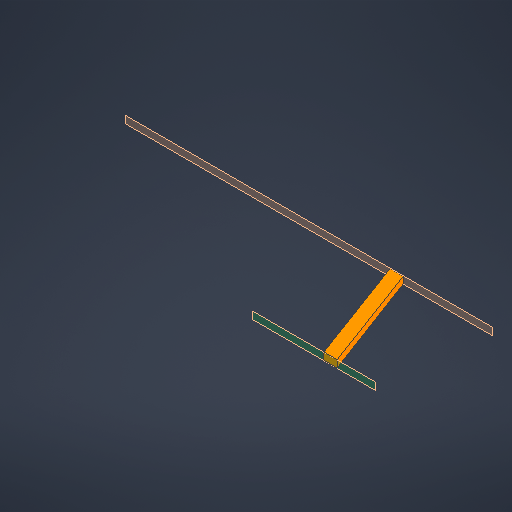
# Autodesk Inventor part: Renamev2
Saved by Autodesk Inventor 2027 (Build 310192000, 192)
## iProperties
Created: 2026-08-07
Part Number: Renamev2
Material: Generic
Document SubType Name: Modeling
Designer: lucas
Density: 1 g/cm^3
Appearance: Default
Author: lucas
Autodesk Inventor part; units mm, degrees
ref_plane "YZ Plane" through (0, 0, 0) normal (1, 0, 0) x (0, 1, 0)
ref_plane "XZ Plane" through (0, 0, 0) normal (0, 1, 0) x (-1, 0, 0)
ref_plane "XY Plane" through (0, 0, 0) normal (0, 0, 1) x (1, 0, 0)
ref_plane "Work Plane1" through (0, 0, 0) normal (0, 0, 1) x (1, 0, 0)
sketch "Sketch1" plane through (0, 0, 0) normal (0, 0, 1) x (1, 0, 0)
  line L0 (1701.8, 0) -> (1701.8, 50.8) projected
  line L1 (1905, 50.5151) -> (2006.6, 50.5151)
  line L2 (2006.6, 50.5151) -> (2006.6, 0)
  line L3 (2006.6, 0) -> (1905, 0)
  line L4 (1905, 0) -> (1905, 50.5151)
  point P0 (0, 0)
  dimension "d0" = 101.6
  dimension "d1" = 203.2
  constraints: 8 end point, 2 parallel, 1 horizontal, 1 perpendicular
  measures "d0" distance of L2.end L3.end
  measures "d1" distance of L0.end L1.start
ref_plane "Work Plane2" through (1701.8, 0, 812.8) normal (0, 0, -1) x (0, 1, 0)
sketch "Sketch2" plane through (1701.8, 0, 812.8) normal (0, 0, -1) x (0, 1, 0)
  line L0 (0, 0) -> (50.8, 0) projected
  line L1 (55.0101, 508) -> (0, 508)
  line L2 (0, 508) -> (0, 609.6)
  line L3 (0, 609.6) -> (55.0101, 609.6)
  line L4 (55.0101, 609.6) -> (55.0101, 508)
  point P0 (0, -1701.8)
  dimension "d2" = 101.6
  dimension "d3" = 609.6
  constraints: 8 end point, 2 parallel, 1 horizontal, 1 perpendicular
  measures "d2" distance of L1.end L2.end
  measures "d3" vertical distance of L0.end L3.end
loft "Loft1" add profiles "Sketch1", "Sketch2"
body "Solid1"
